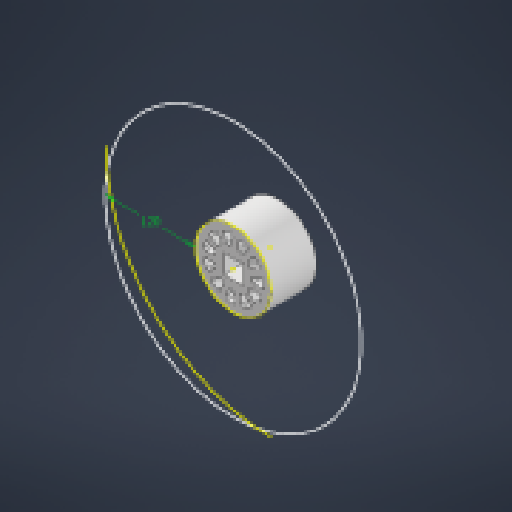
# Autodesk Inventor part: СИСЬКА
Saved by Autodesk Inventor 2025 (Build 290162000, 162)
## iProperties
Created: 2025-10-03
Part Number: СИСЬКА
Material: Типовые
Document SubType Name: Modeling
Designer: Phantom
Density: 1 g/cm^3
Appearance: По умолчанию
Author: Phantom
Autodesk Inventor part; units mm, degrees
ref_plane "YZ Plane" through (0, 0, 0) normal (1, 0, 0) x (0, 1, 0)
ref_plane "XZ Plane" through (0, 0, 0) normal (0, 1, 0) x (-1, 0, 0)
ref_plane "XY Plane" through (0, 0, 0) normal (0, 0, 1) x (1, 0, 0)
sketch "Эскиз1" plane through (0, 0, 0) normal (0, 0, 1) x (1, 0, 0)
  line L0 (-12.5086, -12.3873) -> (-12.5086, 12.6127)
  line L1 (-12.5086, 12.6127) -> (12.4914, 12.6127)
  line L2 (12.4914, 12.6127) -> (12.4914, -12.3873)
  line L3 (12.4914, -12.3873) -> (-12.5086, -12.3873)
  arc A0 (19.9009, 31.4953) -> (19.132, 35.2359) centre (17.9357, 33.0407) ccw
  line L4 (13.5343, 23.3995) -> (19.9009, 31.4953)
  arc A1 (10.5127, 22.679) -> (13.5343, 23.3995) centre (11.5691, 24.9449) ccw
  arc A2 (10.5127, 22.679) -> (7.9494, 23.7053) centre (-0.0086, 0.1127) ccw
  arc A3 (6.2597, 26.3118) -> (7.9494, 23.7053) centre (8.7484, 26.0741) ccw
  line L5 (7.2387, 36.5644) -> (6.2597, 26.3118)
  arc A4 (10.3765, 38.7411) -> (7.2387, 36.5644) centre (9.7274, 36.3268) ccw
  arc A5 (10.3765, 38.7411) -> (-2.8955, 40.0084) centre (-0.0086, 0.1127) ccw
  arc A6 (-0.2264, 37.2773) -> (-2.8955, 40.0084) centre (-2.7151, 37.5149) ccw
  line L6 (-1.2054, 27.0246) -> (-0.2264, 37.2773)
  arc A7 (-3.3578, 24.785) -> (-1.2054, 27.0246) centre (-3.6941, 27.2622) ccw
  arc A8 (-3.3578, 24.785) -> (-6.069, 24.2624) centre (-0.0086, 0.1127) ccw
  arc A9 (-8.8996, 25.5416) -> (-6.069, 24.2624) centre (-6.6775, 26.6872) ccw
  line L7 (-13.619, 34.696) -> (-8.8996, 25.5416)
  arc A10 (-12.1562, 38.2235) -> (-13.619, 34.696) centre (-11.397, 35.8416) ccw
  arc A11 (-12.1562, 38.2235) -> (-24.0064, 32.1143) centre (-0.0086, 0.1127) ccw
  arc A12 (-20.2845, 31.2598) -> (-24.0064, 32.1143) centre (-22.5066, 30.1142) ccw
  line L8 (-15.5651, 22.1054) -> (-20.2845, 31.2598)
  arc A13 (-16.1649, 19.0576) -> (-15.5651, 22.1054) centre (-17.7872, 20.9598) ccw
  arc A14 (-16.1649, 19.0576) -> (-18.1633, 17.1522) centre (-0.0086, 0.1127) ccw
  arc A15 (-21.2361, 16.698) -> (-18.1633, 17.1522) centre (-19.9861, 18.8631) ccw
  line L9 (-30.1556, 21.8477) -> (-21.2361, 16.698)
  arc A16 (-30.8321, 25.6061) -> (-30.1556, 21.8477) centre (-28.9056, 24.0127) ccw
  arc A17 (-30.8321, 25.6061) -> (-37.4982, 14.0599) centre (-0.0086, 0.1127) ccw
  arc A18 (-33.9051, 15.3533) -> (-37.4982, 14.0599) centre (-35.1551, 13.1882) ccw
  line L10 (-24.9857, 10.2036) -> (-33.9051, 15.3533)
  arc A19 (-23.8426, 7.3154) -> (-24.9857, 10.2036) centre (-26.2357, 8.0386) ccw
  arc A20 (-23.8426, 7.3154) -> (-24.4935, 4.6321) centre (-0.0086, 0.1127) ccw
  arc A21 (-26.833, 2.5887) -> (-24.4935, 4.6321) centre (-26.952, 5.0858) ccw
  line L11 (-37.1207, 2.0986) -> (-26.833, 2.5887)
  arc A22 (-39.7217, 4.8947) -> (-37.1207, 2.0986) centre (-37.2396, 4.5958) ccw
  arc A23 (-39.7217, 4.8947) -> (-39.0873, -8.4226) centre (-0.0086, 0.1127) ccw
  arc A24 (-36.7639, -5.392) -> (-39.0873, -8.4226) centre (-36.6449, -7.8891) ccw
  line L12 (-26.4762, -4.9019) -> (-36.7639, -5.392)
  arc A25 (-23.9531, -6.7137) -> (-26.4762, -4.9019) centre (-26.3573, -7.3991) ccw
  arc A26 (-23.9531, -6.7137) -> (-23.05, -9.3229) centre (-0.0086, 0.1127) ccw
  arc A27 (-23.9134, -12.3068) -> (-23.05, -9.3229) centre (-25.3635, -10.2703) ccw
  line L13 (-32.3029, -18.281) -> (-23.9134, -12.3068)
  arc A28 (-36.0027, -17.335) -> (-32.3029, -18.281) centre (-33.7531, -16.2445) ccw
  arc A29 (-36.0027, -17.335) -> (-28.2692, -28.1952) centre (-0.0086, 0.1127) ccw
  arc A30 (-27.9531, -24.3895) -> (-28.2692, -28.1952) centre (-26.5029, -26.426) ccw
  line L14 (-19.5635, -18.4153) -> (-27.9531, -24.3895)
  arc A31 (-16.4614, -18.5754) -> (-19.5635, -18.4153) centre (-18.1133, -20.4518) ccw
  arc A32 (-16.4614, -18.5754) -> (-14.291, -20.2822) centre (-0.0086, 0.1127) ccw
  arc A33 (-13.4041, -23.2591) -> (-14.291, -20.2822) centre (-15.725, -22.33) ccw
  line L15 (-17.232, -32.8207) -> (-13.4041, -23.2591)
  arc A34 (-20.8558, -34.0251) -> (-17.232, -32.8207) centre (-19.5529, -31.8915) ccw
  arc A35 (-20.8558, -34.0251) -> (-8.4785, -38.9803) centre (-0.0086, 0.1127) ccw
  arc A36 (-10.2701, -35.6078) -> (-8.4785, -38.9803) centre (-7.9491, -36.537) ccw
  line L16 (-6.4422, -26.0463) -> (-10.2701, -35.6078)
  arc A37 (-3.746, -24.5037) -> (-6.4422, -26.0463) centre (-4.1213, -26.9754) ccw
  arc A38 (-3.746, -24.5037) -> (-0.9974, -24.7662) centre (-0.0086, 0.1127) ccw
  arc A39 (1.3582, -26.7911) -> (-0.9974, -24.7662) centre (-1.0967, -27.2642) ccw
  line L17 (3.3073, -36.9043) -> (1.3582, -26.7911)
  arc A40 (0.9099, -39.8768) -> (3.3073, -36.9043) centre (0.8525, -37.3774) ccw
  arc A41 (0.9099, -39.8768) -> (14.0013, -37.3536) centre (-0.0086, 0.1127) ccw
  arc A42 (10.6709, -35.4851) -> (14.0013, -37.3536) centre (13.1257, -35.012) ccw
  line L18 (8.7236, -25.3817) -> (10.6709, -35.4851)
  arc A43 (10.1484, -22.6306) -> (8.7236, -25.3817) centre (11.1784, -24.9086) ccw
  arc A44 (10.1484, -22.6306) -> (12.6075, -21.354) centre (-0.397, 0.6896) ccw
  arc A45 (15.6872, -21.782) -> (12.6075, -21.354) centre (13.8778, -23.5072) ccw
  line L19 (22.7938, -29.2353) -> (15.6872, -21.782)
  arc A46 (22.384, -33.032) -> (22.7938, -29.2353) centre (20.9845, -30.9605) ccw
  arc A47 (22.384, -33.032) -> (32.0331, -23.8316) centre (-0.0086, 0.1127) ccw
  arc A48 (28.2212, -24.0603) -> (32.0331, -23.8316) centre (30.0305, -22.3351) ccw
  line L20 (21.1138, -16.6064) -> (28.2212, -24.0603)
  arc A49 (20.8307, -13.513) -> (21.1138, -16.6064) centre (22.9232, -14.8812) ccw
  arc A50 (20.8307, -13.513) -> (22.2113, -11.1218) centre (-0.0086, 0.1127) ccw
  arc A51 (25.0317, -9.8203) -> (22.2113, -11.1218) centre (24.4423, -12.2498) ccw
  line L21 (35.0407, -12.2485) -> (25.0317, -9.8203)
  arc A52 (36.7487, -15.664) -> (35.0407, -12.2485) centre (34.4513, -14.678) ccw
  arc A53 (36.7487, -15.664) -> (39.8919, -2.7075) centre (-0.0086, 0.1127) ccw
  arc A54 (36.8087, -4.9608) -> (39.8919, -2.7075) centre (37.3981, -2.5313) ccw
  line L22 (26.7997, -2.5326) -> (36.8087, -4.9608)
  arc A55 (24.8892, -0.0834) -> (26.7997, -2.5326) centre (27.3891, -0.1031) ccw
  arc A56 (24.8892, -0.0834) -> (24.7578, 2.6746) centre (-0.0086, 0.1127) ccw
  arc A57 (26.4269, 5.2943) -> (24.7578, 2.6746) centre (27.2445, 2.9318) ccw
  line L23 (36.1597, 8.6629) -> (26.4269, 5.2943)
  arc A58 (39.4431, 6.7129) -> (36.1597, 8.6629) centre (36.9774, 6.3004) ccw
  arc A59 (39.4431, 6.7129) -> (29.0156, 27.6372) centre (-0.0086, 0.1127) ccw
  arc A60 (33.6824, 15.9769) -> (35.2772, 18.9519) centre (32.8543, 18.3358) ccw
  line L24 (23.9646, 12.5653) -> (33.6824, 15.9769)
  arc A61 (21.0287, 13.5798) -> (23.9646, 12.5653) centre (23.1364, 14.9241) ccw
  arc A62 (21.0287, 13.5798) -> (19.4171, 15.8219) centre (0.0364, 0.191) ccw
  arc A63 (19.3911, 18.928) -> (19.4171, 15.8219) centre (21.3631, 17.3913) ccw
  line L25 (25.7218, 27.0519) -> (19.3911, 18.928)
  arc A64 (29.0156, 27.6372) -> (25.7218, 27.0519) centre (27.6938, 25.5152) ccw
  arc A65 (29.0156, 27.6372) -> (19.132, 35.2359) centre (-0.0086, 0.1127) ccw
  arc A66 (10.5127, 22.679) -> (7.9494, 23.7053) centre (-0.0086, 0.1127) ccw
  arc A67 (10.5127, 22.679) -> (13.5343, 23.3995) centre (11.5691, 24.9449) ccw
  line L26 (13.5343, 23.3995) -> (19.9009, 31.4953)
  arc A68 (19.9009, 31.4953) -> (19.132, 35.2359) centre (17.9357, 33.0407) ccw
  arc A69 (19.132, 35.2359) -> (10.3765, 38.7411) centre (-0.0086, 0.1127) ccw
  arc A70 (10.3765, 38.7411) -> (7.2387, 36.5644) centre (9.7274, 36.3268) ccw
  line L27 (7.2387, 36.5644) -> (6.2597, 26.3118)
  arc A71 (6.2597, 26.3118) -> (7.9494, 23.7053) centre (8.7484, 26.0741) ccw
  line L28 (-1.2054, 27.0246) -> (-0.2264, 37.2773)
  arc A72 (-0.2264, 37.2773) -> (-2.8955, 40.0084) centre (-2.7151, 37.5149) ccw
  arc A73 (-2.8955, 40.0084) -> (-12.1562, 38.2235) centre (-0.0086, 0.1127) ccw
  arc A74 (-12.1562, 38.2235) -> (-13.619, 34.696) centre (-11.397, 35.8416) ccw
  line L29 (-13.619, 34.696) -> (-8.8996, 25.5416)
  arc A75 (-8.8996, 25.5416) -> (-6.069, 24.2624) centre (-6.6775, 26.6872) ccw
  arc A76 (-3.3578, 24.785) -> (-6.069, 24.2624) centre (-0.0086, 0.1127) ccw
  arc A77 (-3.3578, 24.785) -> (-1.2054, 27.0246) centre (-3.6941, 27.2622) ccw
  circle A78 centre (-22.617, 24.0637) radius 3.1
  arc A79 (-16.1649, 19.0576) -> (-18.1633, 17.1522) centre (-0.0086, 0.1127) ccw
  arc A80 (-16.1649, 19.0576) -> (-15.5651, 22.1054) centre (-17.7872, 20.9598) ccw
  line L30 (-15.5651, 22.1054) -> (-20.2845, 31.2598)
  arc A81 (-20.2845, 31.2598) -> (-24.0064, 32.1143) centre (-22.5066, 30.1142) ccw
  arc A82 (-24.0064, 32.1143) -> (-30.8321, 25.6061) centre (-0.0086, 0.1127) ccw
  arc A83 (-30.8321, 25.6061) -> (-30.1556, 21.8477) centre (-28.9056, 24.0127) ccw
  line L31 (-30.1556, 21.8477) -> (-21.2361, 16.698)
  arc A84 (-21.2361, 16.698) -> (-18.1633, 17.1522) centre (-19.9861, 18.8631) ccw
  arc A85 (-37.4982, 14.0599) -> (-39.7217, 4.8947) centre (-0.0086, 0.1127) ccw
  arc A86 (-39.7217, 4.8947) -> (-37.1207, 2.0986) centre (-37.2396, 4.5958) ccw
  line L32 (-37.1207, 2.0986) -> (-26.833, 2.5887)
  arc A87 (-26.833, 2.5887) -> (-24.4935, 4.6321) centre (-26.952, 5.0858) ccw
  arc A88 (-23.8426, 7.3154) -> (-24.4935, 4.6321) centre (-0.0086, 0.1127) ccw
  arc A89 (-23.8426, 7.3154) -> (-24.9857, 10.2036) centre (-26.2357, 8.0386) ccw
  line L33 (-24.9857, 10.2036) -> (-33.9051, 15.3533)
  arc A90 (-33.9051, 15.3533) -> (-37.4982, 14.0599) centre (-35.1551, 13.1882) ccw
  arc A91 (-39.0873, -8.4226) -> (-36.0027, -17.335) centre (-0.0086, 0.1127) ccw
  arc A92 (-36.0027, -17.335) -> (-32.3029, -18.281) centre (-33.7531, -16.2445) ccw
  line L34 (-32.3029, -18.281) -> (-23.9134, -12.3068)
  arc A93 (-23.9134, -12.3068) -> (-23.05, -9.3229) centre (-25.3635, -10.2703) ccw
  arc A94 (-23.9531, -6.7137) -> (-23.05, -9.3229) centre (-0.0086, 0.1127) ccw
  arc A95 (-23.9531, -6.7137) -> (-26.4762, -4.9019) centre (-26.3573, -7.3991) ccw
  line L35 (-26.4762, -4.9019) -> (-36.7639, -5.392)
  arc A96 (-36.7639, -5.392) -> (-39.0873, -8.4226) centre (-36.6449, -7.8891) ccw
  arc A97 (-8.4785, -38.9803) -> (0.9099, -39.8768) centre (-0.0086, 0.1127) ccw
  arc A98 (0.9099, -39.8768) -> (3.3073, -36.9043) centre (0.8525, -37.3774) ccw
  line L36 (3.3073, -36.9043) -> (1.3582, -26.7911)
  arc A99 (1.3582, -26.7911) -> (-0.9974, -24.7662) centre (-1.0967, -27.2642) ccw
  arc A100 (-3.746, -24.5037) -> (-0.9974, -24.7662) centre (-0.0086, 0.1127) ccw
  arc A101 (-3.746, -24.5037) -> (-6.4422, -26.0463) centre (-4.1213, -26.9754) ccw
  line L37 (-6.4422, -26.0463) -> (-10.2701, -35.6078)
  arc A102 (-10.2701, -35.6078) -> (-8.4785, -38.9803) centre (-7.9491, -36.537) ccw
  arc A103 (14.0013, -37.3536) -> (22.384, -33.032) centre (-0.0086, 0.1127) ccw
  arc A104 (22.384, -33.032) -> (22.7938, -29.2353) centre (20.9845, -30.9605) ccw
  line L38 (22.7938, -29.2353) -> (15.6872, -21.782)
  arc A105 (15.6872, -21.782) -> (12.6075, -21.354) centre (13.8778, -23.5072) ccw
  arc A106 (10.1484, -22.6306) -> (12.6075, -21.354) centre (-0.397, 0.6896) ccw
  arc A107 (10.1484, -22.6306) -> (8.7236, -25.3817) centre (11.1784, -24.9086) ccw
  line L39 (8.7236, -25.3817) -> (10.6709, -35.4851)
  arc A108 (10.6709, -35.4851) -> (14.0013, -37.3536) centre (13.1257, -35.012) ccw
  circle A109 centre (-20.4983, -25.6742) radius 3.1
  arc A110 (-28.2692, -28.1952) -> (-20.8558, -34.0251) centre (-0.0086, 0.1127) ccw
  arc A111 (-20.8558, -34.0251) -> (-17.232, -32.8207) centre (-19.5529, -31.8915) ccw
  line L40 (-17.232, -32.8207) -> (-13.4041, -23.2591)
  arc A112 (-13.4041, -23.2591) -> (-14.291, -20.2822) centre (-15.725, -22.33) ccw
  arc A113 (-16.4614, -18.5754) -> (-14.291, -20.2822) centre (-0.0086, 0.1127) ccw
  arc A114 (-16.4614, -18.5754) -> (-19.5635, -18.4153) centre (-18.1133, -20.4518) ccw
  line L41 (-19.5635, -18.4153) -> (-27.9531, -24.3895)
  arc A115 (-27.9531, -24.3895) -> (-28.2692, -28.1952) centre (-26.5029, -26.426) ccw
  arc A116 (20.8307, -13.513) -> (22.2113, -11.1218) centre (-0.0086, 0.1127) ccw
  arc A117 (20.8307, -13.513) -> (21.1138, -16.6064) centre (22.9232, -14.8812) ccw
  line L42 (21.1138, -16.6064) -> (28.2212, -24.0603)
  arc A118 (28.2212, -24.0603) -> (32.0331, -23.8316) centre (30.0305, -22.3351) ccw
  arc A119 (32.0331, -23.8316) -> (36.7487, -15.664) centre (-0.0086, 0.1127) ccw
  arc A120 (36.7487, -15.664) -> (35.0407, -12.2485) centre (34.4513, -14.678) ccw
  line L43 (35.0407, -12.2485) -> (25.0317, -9.8203)
  arc A121 (25.0317, -9.8203) -> (22.2113, -11.1218) centre (24.4423, -12.2498) ccw
  circle A122 centre (32.8977, 1.5144) radius 3.1
  line L44 (26.7997, -2.5326) -> (36.8087, -4.9608)
  arc A123 (36.8087, -4.9608) -> (39.8919, -2.7075) centre (37.3981, -2.5313) ccw
  arc A124 (39.8919, -2.7075) -> (39.4431, 6.7129) centre (-0.0086, 0.1127) ccw
  arc A125 (39.4431, 6.7129) -> (36.1597, 8.6629) centre (36.9774, 6.3004) ccw
  line L45 (36.1597, 8.6629) -> (26.4269, 5.2943)
  arc A126 (26.4269, 5.2943) -> (24.7578, 2.6746) centre (27.2445, 2.9318) ccw
  arc A127 (24.8892, -0.0834) -> (24.7578, 2.6746) centre (-0.0086, 0.1127) ccw
  arc A128 (24.8892, -0.0834) -> (26.7997, -2.5326) centre (27.3891, -0.1031) ccw
  circle A129 centre (-0.0086, 0.1127) radius 50
  point P0 (0, 0)
  point P1 (-1.5277, -0.5383)
  point P2 (19.132, 35.2359)
  point P3 (6.2597, 26.3118)
  point P4 (-2.8955, 40.0084)
  point P5 (-6.069, 24.2624)
  point P6 (-8.8996, 25.5416)
  point P7 (-12.1562, 38.2235)
  point P8 (-21.2361, 16.698)
  point P9 (-39.7217, 4.8947)
  point P10 (-39.0873, -8.4226)
  point P11 (-36.0027, -17.335)
  point P12 (-28.2692, -28.1952)
  point P13 (-8.4785, -38.9803)
  point P14 (0.9099, -39.8768)
  point P15 (14.0013, -37.3536)
  point P16 (22.384, -33.032)
  point P17 (26.7997, -2.5326)
  dimension "d0" = 100
  constraints: 253 point on circle, 130 centre point, 92 end point, 1 coincident
  measures "d0" diameter of A129
extrude "Выдавливание1" add sketch "Эскиз1" along normal blind 60 contours A0 A65 A64 L25 A63 A62 A61 L24 A60 A59 A58 L23 A57 A56 A55 L22 A54 A53 A52 L21 A51 A50 A49 L20 A48 A47 A46 L19 A45 A44 A43 L18 A42 A41 A40 L17 A39 A38 A37 L16 A36 A35 A34 L15 A33 A32 A31 L14 A30 A29 A28 L13 A27 A26 A25 L12 A24 A23 A22 L11 A21 A20 A19 L10 A18 A17 A16 L9 A15 A14 A13 L8 A12 A11 A10 L7 A9 A8 A7 L6 A6 A5 A4 L5 A3 A2 A1 L4 | A129
